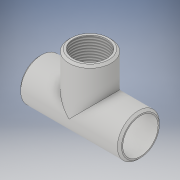
# Autodesk Inventor part: penyambung
Saved by Autodesk Inventor 2019.5 (Build 235369000, 369)
## iProperties
Created: 2022-10-10
Part Number: penyambung
Material: Generic
Document SubType Name: Modeling
Designer: ASUS
Density: 1 g/cm^3
Appearance: Default
Author: ASUS
Autodesk Inventor part; units mm, degrees
ref_plane "YZ Plane" through (0, 0, 0) normal (1, 0, 0) x (0, 1, 0)
ref_plane "XZ Plane" through (0, 0, 0) normal (0, 1, 0) x (-1, 0, 0)
ref_plane "XY Plane" through (0, 0, 0) normal (0, 0, 1) x (1, 0, 0)
sketch "Sketch2" plane through (0, 0, 0) normal (0, 0, 1) x (1, 0, 0)
  line L0 (60, 0) -> (60, 60)
  line L1 (0, 0) -> (0, -25)
  line L2 (0, -25) -> (120, -25)
  line L3 (120, -25) -> (120, 0)
  line L4 (60, 60) -> (85, 60)
  line L5 (85, 60) -> (85, 0)
  line L6 (60, 0) -> (85, 0)
  line L7 (0, 0) -> (120, 0)
  dimension "d4" = 120
  dimension "d5" = 60
  dimension "d6" = 25
  dimension "d7" = 25
  constraints: 16 end point, 3 perpendicular, 2 vertical, 1 horizontal
  measures "d4" distance of L1.start L3.end
  measures "d5" distance of L0.start L0.end
  measures "d6" distance of L1.start L1.end
  measures "d7" distance of L0.end L4.end
revolve "Revolution1" add sketch "Sketch2" angle 360 about axis through (0, 0, 0) along (1, 0, 0) contours L6 L7 L3 L2 L1
revolve "Revolution2" add sketch "Sketch2" angle 360 about axis through (60, 0, 0) along (0, 1, 0) contours L0 L4 L5 L6
sketch "Sketch3" plane through (60, 60, 0) normal (0, 1, 0) x (1, 0, 0)
  point P0 (-60, 0)
  point P1 (0.0519, -0.0386)
hole "Hole1" at (60.0519, 60, 0.0386) direction (0, -1, 0) diameter 40 depth 35
shell "Shell1" thickness 4 removed faces 2 at (120, -4.976, 4.8639) at (0, 0.7623, 6.2783)
chamfer "Chamfer1" distance 2.5 angle 45 3 edges at (0, 25, 0) (120, 25, 0) (35, 60, 0)
thread "Thread1" size "M40x3" class "6H" standard "ANSI Metric M Profile" full length
body "Solid1"
